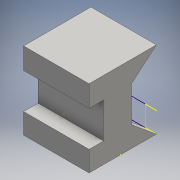
# Autodesk Inventor part: 240510_3Dsketch09
Saved by Autodesk Inventor 2016 (Build 200138000, 138)
## iProperties
Created: 2024-05-10
Part Number: 240510_3Dsketch09
Material: 일반
Document SubType Name: Modeling
Designer: pc
Density: 1 g/cm^3
Appearance: 기본값
Author: pc
Autodesk Inventor part; units mm, degrees
ref_plane "YZ Plane" through (0, 0, 0) normal (1, 0, 0) x (0, 1, 0)
ref_plane "XZ Plane" through (0, 0, 0) normal (0, 1, 0) x (-1, 0, 0)
ref_plane "XY Plane" through (0, 0, 0) normal (0, 0, 1) x (1, 0, 0)
sketch "스케치1" plane through (0, 0, 0) normal (0, 0, 1) x (1, 0, 0)
  line L0 (-9.8208, 11.7001) -> (11.3566, 11.7001)
  line L1 (11.3566, 11.7001) -> (11.3566, -10.0835)
  line L2 (11.3566, -10.0835) -> (-9.8208, -10.0835)
  line L3 (-9.8208, -10.0835) -> (-9.8208, 11.7001)
  point P0 (0, 0)
  constraints: 8 end point, 2 parallel, 1 horizontal, 1 perpendicular
extrude "돌출1" add sketch "스케치1" along normal blind 25
sketch "스케치2" plane through (11.3566, -10.0835, 0) normal (1, 0, 0) x (0, 0, -1)
  line L0 (0, 0) -> (-25, 0) projected
  line L1 (-18.1058, 4.6881) -> (-6.628, 4.6881)
  line L2 (-6.628, 4.6881) -> (-6.628, 0)
  line L3 (-6.628, 0) -> (-18.1058, 0)
  line L4 (-18.1058, 0) -> (-18.1058, 4.6881)
  point P0 (0, 10.0835)
  constraints: 8 end point, 2 parallel, 1 horizontal, 1 perpendicular, 1 point on line
extrude "돌출2" cut sketch "스케치2" against normal blind 25
sketch "스케치3" plane through (11.3566, -10.0835, 0) normal (1, 0, 0) x (0, 0, -1)
  line L0 (0, 21.7836) -> (-25, 21.7836) projected
  line L1 (-18.1058, 21.7836) -> (-6.6684, 21.7836)
  line L2 (-6.6684, 21.7836) -> (-6.6684, 13.7006)
  line L3 (-6.6684, 13.7006) -> (-18.1058, 13.7006)
  line L4 (-18.1058, 13.7006) -> (-18.1058, 21.7836)
  point P0 (0, 10.0835)
  constraints: 8 end point, 2 parallel, 1 horizontal, 1 perpendicular, 1 point on line
extrude "돌출3" cut sketch "스케치3" against normal blind 25
sketch "스케치4" plane through (11.3566, -10.0835, 0) normal (1, 0, 0) x (0, 0, -1)
  point P0 (0, 10.0835)
sketch "스케치5" plane through (-9.8208, 11.7001, 0) normal (0, 1, 0) x (1, 0, 0)
  line L0 (21.1774, -6.628) -> (0, -6.628) projected
  line L1 (0, 0) -> (21.1774, 0) projected
  line L2 (4.1053, -6.628) -> (17.5214, -6.628)
  line L3 (17.5214, -6.628) -> (17.5214, 0)
  line L4 (17.5214, 0) -> (4.1053, 0)
  line L5 (4.1053, 0) -> (4.1053, -6.628)
  point P0 (9.8208, 0)
  constraints: 8 end point, 2 parallel, 2 point on line, 1 horizontal, 1 perpendicular
sketch "스케치6" plane through (11.3566, 3.6171, 6.6684) normal (0, 0, 1) x (1, 0, 0)
  line L0 (-21.1774, 8.083) -> (0, 8.083) projected
  line L1 (0, 0) -> (-21.1774, 0) projected
  line L2 (-16.9228, 8.083) -> (-3.828, 8.083)
  line L3 (-3.828, 8.083) -> (-3.828, 0)
  line L4 (-3.828, 0) -> (-16.9228, 0)
  line L5 (-16.9228, 0) -> (-16.9228, 8.083)
  point P0 (-11.3566, -3.6171)
  constraints: 8 end point, 2 parallel, 2 point on line, 1 horizontal, 1 perpendicular
extrude "돌출4" cut sketch "스케치6" against normal blind 10
sketch "스케치7" plane through (11.3566, -10.0835, 0) normal (1, 0, 0) x (0, 0, -1)
  line L0 (-6.6684, 13.7006) -> (-18.1058, 13.7006) projected
  line L1 (0, 21.7836) -> (0, 13.7006) projected
  line L2 (-6.6684, 13.7006) -> (0, 21.7836)
  line L3 (-6.6684, 13.7006) -> (-6.6684, 21.7836)
  line L4 (0, 21.7836) -> (0, 0) projected
  line L5 (-6.6684, 21.7836) -> (0, 21.7836)
  point P0 (0, 10.0835)
  constraints: 6 end point, 1 perpendicular, 1 vertical
extrude "돌출5" cut sketch "스케치7" against normal blind 50
sketch "스케치8" plane through (11.3566, -10.0835, 25) normal (1, 0, 0) x (0, 0, -1)
  line L0 (0, 21.7836) -> (0, 0) projected
  line L1 (6.8942, 13.7006) -> (18.3316, 13.7006) projected
  line L2 (0, 21.7836) -> (6.8942, 13.7006)
  line L3 (6.8942, 21.7836) -> (6.8942, 13.7006) projected
  line L4 (6.8942, 13.7006) -> (6.8942, 21.7836)
  line L5 (6.8942, 21.7836) -> (0, 21.7836) projected
  line L6 (6.8942, 21.7836) -> (0, 21.7836)
  point P0 (25, 10.0835)
  constraints: 6 end point, 2 collinear
extrude "돌출6" cut sketch "스케치8" against normal blind 15
